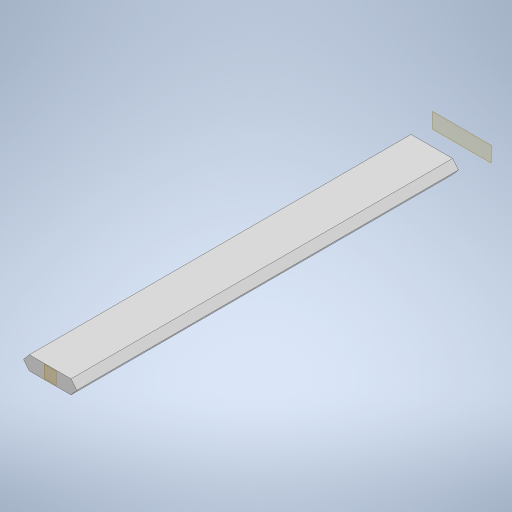
# Autodesk Inventor part: Enemy_gun_collision
Saved by Autodesk Inventor 2024 (Build 280153000, 153)
## iProperties
Created: 2026-05-20
Part Number: Enemy_gun_collision
Material: Generic
Document SubType Name: Modeling
Designer: warny
Density: 1 g/cm^3
Appearance: Default
Author: warny
Autodesk Inventor part; units mm, degrees
ref_plane "YZ Plane" through (0, 0, 0) normal (1, 0, 0) x (0, 1, 0)
ref_plane "XZ Plane" through (0, 0, 0) normal (0, 1, 0) x (-1, 0, 0)
ref_plane "Work Plane1" through (0, 0, 672.2) normal (0, 0, 1) x (1, 0, 0)
sketch "Sketch1" plane through (0, 0, 672.2) normal (0, 0, 1) x (1, 0, 0)
  line L0 (0, -15.96) -> (0, 15.96) projected
  line L1 (0, 11.4) -> (34, 11.4)
  line L2 (34, 11.4) -> (43.6, 0)
  line L3 (43.6, 0) -> (34, -11.4)
  line L4 (34, -11.4) -> (0, -11.4)
  line L5 (-34, 11.4) -> (0, 11.4)
  line L6 (-61.04, 0) -> (61.04, 0) construction
  line L7 (-34, 11.4) -> (-43.6, 0)
  line L8 (-43.6, 0) -> (-34, -11.4)
  line L9 (-34, -11.4) -> (0, -11.4)
  point P0 (0, 0)
  dimension "d1" = 34
  dimension "d2" = 34
  dimension "d3" = 11.4
  dimension "d5" = 43.6
  dimension "d7" = 43.6
  dimension "d8" = 34
  dimension "d9" = 34
  dimension "d10" = 11.4
  constraints: 16 end point, 5 point on line, 2 horizontal, 2 perpendicular
  measures "d1" distance of L1.end L1.start
  measures "d2" distance from line of L0 L5.start
  measures "d3" distance between parallel lines of L6 L5
  measures "d5" distance from line of L0 L2.end
  measures "d7" distance from line of L0 L7.end
  measures "d8" distance of L8.end L4.end
  measures "d9" distance from line of L0 L3.end
  measures "d10" distance from line of L6 L8.end
extrude "Extrusion1" add sketch "Sketch1" against normal blind 623.2
body "Solid1"
